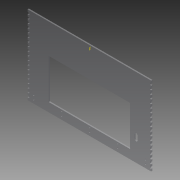
# Autodesk Inventor part: case_front
Saved by Autodesk Inventor 2014 (Build 180170000, 170)
## iProperties
Created: 2013-08-29
Part Number: case_front
Material: Polycarbonate, Clear
Document SubType Name: Modeling
Designer: Edward
Density: 1.2 g/cm^3
Appearance: Polycarbonate - Clear
Author: Edward
Autodesk Inventor part; units mm, degrees
ref_plane "YZ Plane" through (0, 0, 0) normal (1, 0, 0) x (0, 1, 0)
ref_plane "XZ Plane" through (0, 0, 0) normal (0, 1, 0) x (-1, 0, 0)
ref_plane "XY Plane" through (0, 0, 0) normal (0, 0, 1) x (1, 0, 0)
sketch "Sketch1" plane through (0, 0, 0) normal (0, 0, 1) x (1, 0, 0)
  line L0 (303, -45.4136) -> (309.35, -45.4136) projected
  line L1 (303, -45.4136) -> (303, -33.5636) projected
  line L2 (303, 348.2864) -> (309.35, 348.2864) projected
  line L3 (-309.35, 348.2864) -> (-303, 348.2864) projected
  line L4 (-303, -33.5636) -> (-303, -45.4136) projected
  line L5 (303, -45.4136) -> (-303, -45.4136)
  line L6 (-303, -45.4136) -> (-303, 348.2864)
  line L7 (-303, 348.2864) -> (303, 348.2864)
  line L8 (303, 348.2864) -> (303, -45.4136)
  point P0 (0, 0)
  constraints: 8 end point, 2 parallel, 1 horizontal, 1 perpendicular
extrude "Extrusion1" add sketch "Sketch1" along normal blind 6.35
sketch "Sketch3" plane through (303, -45.4136, 0) normal (1, 0, 0) x (0, 0, -1)
  line L0 (0, 393.7) -> (0, 0) projected
  line L1 (-6.35, 0) -> (-6.35, 393.7) projected
  line L2 (0, 21.85) -> (-6.35, 21.85) projected
  line L3 (0, 31.85) -> (-6.35, 31.85) projected
  point P0 (0, 45.4136)
extrude "Extrusion3" add sketch "Sketch3" along normal blind 6.35
pattern_linear "Rectangular Pattern1" count 18 spacing 20 along (0, 1, 0) of "Extrusion3"
sketch "Sketch4" plane through (303, 348.2864, 6.35) normal (1, 0, 0) x (0, 0, -1)
  line L0 (6.35, 0) -> (0, 0) projected
  line L1 (0, -21.85) -> (0, 0) projected
  circle A0 centre (454.35, -377.7) radius 2.75 projected
  circle A1 centre (259.35, -357.7) radius 2.75 projected
  circle A2 centre (64.35, -377.7) radius 2.75 projected
  circle A3 centre (64.35, -357.7) radius 2.75 projected
  circle A4 centre (259.35, -377.7) radius 2.75 projected
  circle A5 centre (454.35, -357.7) radius 2.75 projected
  arc A6 (30.35, -355.2) -> (18.35, -355.2) centre (24.35, -355.2) ccw projected
  line L2 (30.35, -355.2) -> (30.35, -380.2) projected
  arc A7 (18.35, -380.2) -> (30.35, -380.2) centre (24.35, -380.2) ccw projected
  line L3 (18.35, -380.2) -> (18.35, -355.2) projected
  arc A8 (488.35, -380.2) -> (500.35, -380.2) centre (494.35, -380.2) ccw projected
  line L4 (488.35, -380.2) -> (488.35, -355.2) projected
  arc A9 (500.35, -355.2) -> (488.35, -355.2) centre (494.35, -355.2) ccw projected
  line L5 (500.35, -355.2) -> (500.35, -380.2) projected
  line L6 (6.35, -393.7) -> (512.35, -393.7) projected
  line L7 (512.35, -393.7) -> (512.35, -381.85) projected
  line L8 (512.35, -381.85) -> (518.7, -381.85) projected
  line L9 (518.7, -371.85) -> (518.7, -381.85) projected
  line L10 (512.35, -371.85) -> (518.7, -371.85) projected
  line L11 (512.35, -371.85) -> (512.35, -361.85) projected
  line L12 (512.35, -361.85) -> (518.7, -361.85) projected
  line L13 (518.7, -351.85) -> (518.7, -361.85) projected
  line L14 (512.35, -351.85) -> (518.7, -351.85) projected
  line L15 (512.35, -351.85) -> (512.35, -341.85) projected
  line L16 (512.35, -341.85) -> (518.7, -341.85) projected
  line L17 (518.7, -331.85) -> (518.7, -341.85) projected
  line L18 (512.35, -331.85) -> (518.7, -331.85) projected
  line L19 (512.35, -331.85) -> (512.35, -321.85) projected
  line L20 (512.35, -321.85) -> (518.7, -321.85) projected
  line L21 (518.7, -311.85) -> (518.7, -321.85) projected
  line L22 (512.35, -311.85) -> (518.7, -311.85) projected
  line L23 (512.35, -311.85) -> (512.35, -301.85) projected
  line L24 (512.35, -301.85) -> (518.7, -301.85) projected
  line L25 (518.7, -291.85) -> (518.7, -301.85) projected
  line L26 (512.35, -291.85) -> (518.7, -291.85) projected
  line L27 (512.35, -291.85) -> (512.35, -281.85) projected
  line L28 (512.35, -281.85) -> (518.7, -281.85) projected
  line L29 (518.7, -271.85) -> (518.7, -281.85) projected
  line L30 (512.35, -271.85) -> (518.7, -271.85) projected
  line L31 (512.35, -271.85) -> (512.35, -261.85) projected
  line L32 (512.35, -261.85) -> (518.7, -261.85) projected
  line L33 (518.7, -251.85) -> (518.7, -261.85) projected
  line L34 (512.35, -251.85) -> (518.7, -251.85) projected
  line L35 (512.35, -251.85) -> (512.35, -241.85) projected
  line L36 (512.35, -241.85) -> (518.7, -241.85) projected
  line L37 (518.7, -231.85) -> (518.7, -241.85) projected
  line L38 (512.35, -231.85) -> (518.7, -231.85) projected
  line L39 (512.35, -231.85) -> (512.35, -221.85) projected
  line L40 (512.35, -221.85) -> (518.7, -221.85) projected
  line L41 (518.7, -211.85) -> (518.7, -221.85) projected
  line L42 (512.35, -211.85) -> (518.7, -211.85) projected
  line L43 (512.35, -211.85) -> (512.35, -201.85) projected
  line L44 (512.35, -201.85) -> (518.7, -201.85) projected
  line L45 (518.7, -191.85) -> (518.7, -201.85) projected
  line L46 (512.35, -191.85) -> (518.7, -191.85) projected
  line L47 (512.35, -191.85) -> (512.35, -181.85) projected
  line L48 (512.35, -181.85) -> (518.7, -181.85) projected
  line L49 (518.7, -171.85) -> (518.7, -181.85) projected
  line L50 (512.35, -171.85) -> (518.7, -171.85) projected
  line L51 (512.35, -171.85) -> (512.35, -161.85) projected
  line L52 (512.35, -161.85) -> (518.7, -161.85) projected
  line L53 (518.7, -151.85) -> (518.7, -161.85) projected
  line L54 (512.35, -151.85) -> (518.7, -151.85) projected
  line L55 (512.35, -151.85) -> (512.35, -141.85) projected
  line L56 (512.35, -141.85) -> (518.7, -141.85) projected
  line L57 (518.7, -131.85) -> (518.7, -141.85) projected
  line L58 (512.35, -131.85) -> (518.7, -131.85) projected
  line L59 (512.35, -131.85) -> (512.35, -121.85) projected
  line L60 (512.35, -121.85) -> (518.7, -121.85) projected
  line L61 (518.7, -111.85) -> (518.7, -121.85) projected
  line L62 (512.35, -111.85) -> (518.7, -111.85) projected
  line L63 (512.35, -111.85) -> (512.35, -101.85) projected
  line L64 (512.35, -101.85) -> (518.7, -101.85) projected
  line L65 (518.7, -91.85) -> (518.7, -101.85) projected
  line L66 (512.35, -91.85) -> (518.7, -91.85) projected
  line L67 (512.35, -91.85) -> (512.35, -81.85) projected
  line L68 (512.35, -81.85) -> (518.7, -81.85) projected
  line L69 (518.7, -71.85) -> (518.7, -81.85) projected
  line L70 (512.35, -71.85) -> (518.7, -71.85) projected
  line L71 (512.35, -71.85) -> (512.35, -61.85) projected
  line L72 (512.35, -61.85) -> (518.7, -61.85) projected
  line L73 (518.7, -51.85) -> (518.7, -61.85) projected
  line L74 (512.35, -51.85) -> (518.7, -51.85) projected
  line L75 (512.35, -51.85) -> (512.35, -41.85) projected
  line L76 (512.35, -41.85) -> (518.7, -41.85) projected
  line L77 (518.7, -31.85) -> (518.7, -41.85) projected
  line L78 (512.35, -31.85) -> (518.7, -31.85) projected
  line L79 (512.35, -31.85) -> (512.35, -21.85) projected
  line L80 (512.35, -21.85) -> (518.7, -21.85) projected
  line L81 (518.7, -11.85) -> (518.7, -21.85) projected
  line L82 (512.35, -11.85) -> (518.7, -11.85) projected
  line L83 (512.35, -11.85) -> (512.35, 0) projected
  line L84 (100.7265, 0) -> (90.7265, 0) projected
  line L85 (6.35, 0) -> (6.35, -11.85) projected
  line L86 (6.35, -11.85) -> (0, -11.85) projected
  line L87 (0, -21.85) -> (0, -11.85) projected
  line L88 (6.35, -21.85) -> (0, -21.85) projected
  line L89 (6.35, -21.85) -> (6.35, -31.85) projected
  line L90 (6.35, -31.85) -> (0, -31.85) projected
  line L91 (0, -41.85) -> (0, -31.85) projected
  line L92 (6.35, -41.85) -> (0, -41.85) projected
  line L93 (6.35, -41.85) -> (6.35, -51.85) projected
  line L94 (6.35, -51.85) -> (0, -51.85) projected
  line L95 (0, -61.85) -> (0, -51.85) projected
  line L96 (6.35, -61.85) -> (0, -61.85) projected
  line L97 (6.35, -61.85) -> (6.35, -71.85) projected
  line L98 (6.35, -71.85) -> (0, -71.85) projected
  line L99 (0, -81.85) -> (0, -71.85) projected
  line L100 (6.35, -81.85) -> (0, -81.85) projected
  line L101 (6.35, -81.85) -> (6.35, -91.85) projected
  line L102 (6.35, -91.85) -> (0, -91.85) projected
  line L103 (0, -101.85) -> (0, -91.85) projected
  line L104 (6.35, -101.85) -> (0, -101.85) projected
  line L105 (6.35, -101.85) -> (6.35, -111.85) projected
  line L106 (6.35, -111.85) -> (0, -111.85) projected
  line L107 (0, -121.85) -> (0, -111.85) projected
  line L108 (6.35, -121.85) -> (0, -121.85) projected
  line L109 (6.35, -121.85) -> (6.35, -131.85) projected
  line L110 (6.35, -131.85) -> (0, -131.85) projected
  line L111 (0, -141.85) -> (0, -131.85) projected
  line L112 (6.35, -141.85) -> (0, -141.85) projected
  line L113 (6.35, -141.85) -> (6.35, -151.85) projected
  line L114 (6.35, -151.85) -> (0, -151.85) projected
  line L115 (0, -161.85) -> (0, -151.85) projected
  line L116 (6.35, -161.85) -> (0, -161.85) projected
  line L117 (6.35, -161.85) -> (6.35, -171.85) projected
  line L118 (6.35, -171.85) -> (0, -171.85) projected
  line L119 (0, -181.85) -> (0, -171.85) projected
  line L120 (6.35, -181.85) -> (0, -181.85) projected
  line L121 (6.35, -181.85) -> (6.35, -191.85) projected
  line L122 (6.35, -191.85) -> (0, -191.85) projected
  line L123 (0, -201.85) -> (0, -191.85) projected
  line L124 (6.35, -201.85) -> (0, -201.85) projected
  line L125 (6.35, -201.85) -> (6.35, -211.85) projected
  line L126 (6.35, -211.85) -> (0, -211.85) projected
  line L127 (0, -221.85) -> (0, -211.85) projected
  line L128 (6.35, -221.85) -> (0, -221.85) projected
  line L129 (6.35, -221.85) -> (6.35, -231.85) projected
  line L130 (6.35, -231.85) -> (0, -231.85) projected
  line L131 (0, -241.85) -> (0, -231.85) projected
  line L132 (6.35, -241.85) -> (0, -241.85) projected
  line L133 (6.35, -241.85) -> (6.35, -251.85) projected
  line L134 (6.35, -251.85) -> (0, -251.85) projected
  line L135 (0, -261.85) -> (0, -251.85) projected
  line L136 (6.35, -261.85) -> (0, -261.85) projected
  line L137 (6.35, -261.85) -> (6.35, -271.85) projected
  line L138 (6.35, -271.85) -> (0, -271.85) projected
  line L139 (0, -281.85) -> (0, -271.85) projected
  line L140 (6.35, -281.85) -> (0, -281.85) projected
  line L141 (6.35, -281.85) -> (6.35, -291.85) projected
  line L142 (6.35, -291.85) -> (0, -291.85) projected
  line L143 (0, -301.85) -> (0, -291.85) projected
  line L144 (6.35, -301.85) -> (0, -301.85) projected
  line L145 (6.35, -301.85) -> (6.35, -311.85) projected
  line L146 (6.35, -311.85) -> (0, -311.85) projected
  line L147 (0, -321.85) -> (0, -311.85) projected
  line L148 (6.35, -321.85) -> (0, -321.85) projected
  line L149 (6.35, -321.85) -> (6.35, -331.85) projected
  line L150 (6.35, -331.85) -> (0, -331.85) projected
  line L151 (0, -341.85) -> (0, -331.85) projected
  line L152 (6.35, -341.85) -> (0, -341.85) projected
  line L153 (6.35, -341.85) -> (6.35, -351.85) projected
  line L154 (6.35, -351.85) -> (0, -351.85) projected
  line L155 (0, -361.85) -> (0, -351.85) projected
  line L156 (6.35, -361.85) -> (0, -361.85) projected
  line L157 (6.35, -361.85) -> (6.35, -371.85) projected
  line L158 (6.35, -371.85) -> (0, -371.85) projected
  line L159 (0, -381.85) -> (0, -371.85) projected
  line L160 (6.35, -381.85) -> (0, -381.85) projected
  line L161 (6.35, -381.85) -> (6.35, -393.7) projected
  line L162 (6.35, -393.7) -> (0, -393.7) projected
  line L163 (0, -393.7) -> (0, -371.85) projected
  line L164 (480.7265, -6.35) -> (480.7265, 0) projected
  line L165 (480.7265, 0) -> (470.7265, 0) projected
  line L166 (470.7265, 0) -> (470.7265, -6.35) projected
  line L167 (470.7265, -6.35) -> (460.7265, -6.35) projected
  line L168 (460.7265, -6.35) -> (460.7265, 0) projected
  line L169 (460.7265, 0) -> (450.7265, 0) projected
  line L170 (450.7265, 0) -> (450.7265, -6.35) projected
  line L171 (450.7265, -6.35) -> (440.7265, -6.35) projected
  line L172 (440.7265, -6.35) -> (440.7265, 0) projected
  line L173 (440.7265, 0) -> (430.7265, 0) projected
  line L174 (430.7265, 0) -> (430.7265, -6.35) projected
  line L175 (430.7265, -6.35) -> (420.7265, -6.35) projected
  line L176 (420.7265, -6.35) -> (420.7265, 0) projected
  line L177 (420.7265, 0) -> (410.7265, 0) projected
  line L178 (410.7265, 0) -> (410.7265, -6.35) projected
  line L179 (410.7265, -6.35) -> (400.7265, -6.35) projected
  line L180 (400.7265, -6.35) -> (400.7265, 0) projected
  line L181 (400.7265, 0) -> (390.7265, 0) projected
  line L182 (390.7265, 0) -> (390.7265, -6.35) projected
  line L183 (390.7265, -6.35) -> (380.7265, -6.35) projected
  line L184 (380.7265, -6.35) -> (380.7265, 0) projected
  line L185 (380.7265, 0) -> (370.7265, 0) projected
  line L186 (370.7265, 0) -> (370.7265, -6.35) projected
  line L187 (370.7265, -6.35) -> (360.7265, -6.35) projected
  line L188 (360.7265, -6.35) -> (360.7265, 0) projected
  line L189 (360.7265, 0) -> (350.7265, 0) projected
  line L190 (350.7265, 0) -> (350.7265, -6.35) projected
  line L191 (350.7265, -6.35) -> (340.7265, -6.35) projected
  line L192 (340.7265, -6.35) -> (340.7265, 0) projected
  line L193 (340.7265, 0) -> (330.7265, 0) projected
  line L194 (330.7265, 0) -> (330.7265, -6.35) projected
  line L195 (330.7265, -6.35) -> (320.7265, -6.35) projected
  line L196 (320.7265, -6.35) -> (320.7265, 0) projected
  line L197 (320.7265, 0) -> (310.7265, 0) projected
  line L198 (310.7265, 0) -> (310.7265, -6.35) projected
  line L199 (310.7265, -6.35) -> (300.7265, -6.35) projected
  line L200 (300.7265, -6.35) -> (300.7265, 0) projected
  line L201 (300.7265, 0) -> (290.7265, 0) projected
  line L202 (290.7265, 0) -> (290.7265, -6.35) projected
  line L203 (290.7265, -6.35) -> (280.7265, -6.35) projected
  line L204 (280.7265, -6.35) -> (280.7265, 0) projected
  line L205 (280.7265, 0) -> (270.7265, 0) projected
  line L206 (270.7265, 0) -> (270.7265, -6.35) projected
  line L207 (270.7265, -6.35) -> (260.7265, -6.35) projected
  line L208 (260.7265, -6.35) -> (260.7265, 0) projected
  line L209 (260.7265, 0) -> (250.7265, 0) projected
  line L210 (250.7265, 0) -> (250.7265, -6.35) projected
  line L211 (250.7265, -6.35) -> (240.7265, -6.35) projected
  line L212 (240.7265, -6.35) -> (240.7265, 0) projected
  line L213 (230.7265, 0) -> (230.7265, -6.35) projected
  line L214 (230.7265, -6.35) -> (220.7265, -6.35) projected
  line L215 (220.7265, -6.35) -> (220.7265, 0) projected
  line L216 (220.7265, 0) -> (210.7265, 0) projected
  line L217 (210.7265, 0) -> (210.7265, -6.35) projected
  line L218 (210.7265, -6.35) -> (200.7265, -6.35) projected
  line L219 (200.7265, -6.35) -> (200.7265, 0) projected
  line L220 (200.7265, 0) -> (190.7265, 0) projected
  line L221 (190.7265, 0) -> (190.7265, -6.35) projected
  line L222 (190.7265, -6.35) -> (180.7265, -6.35) projected
  line L223 (180.7265, -6.35) -> (180.7265, 0) projected
  line L224 (180.7265, 0) -> (170.7265, 0) projected
  line L225 (170.7265, 0) -> (170.7265, -6.35) projected
  line L226 (170.7265, -6.35) -> (160.7265, -6.35) projected
  line L227 (160.7265, -6.35) -> (160.7265, 0) projected
  line L228 (160.7265, 0) -> (150.7265, 0) projected
  line L229 (150.7265, 0) -> (150.7265, -6.35) projected
  line L230 (150.7265, -6.35) -> (140.7265, -6.35) projected
  line L231 (140.7265, -6.35) -> (140.7265, 0) projected
  line L232 (140.7265, 0) -> (130.7265, 0) projected
  line L233 (130.7265, 0) -> (130.7265, -6.35) projected
  line L234 (130.7265, -6.35) -> (120.7265, -6.35) projected
  line L235 (120.7265, -6.35) -> (120.7265, 0) projected
  line L236 (120.7265, 0) -> (110.7265, 0) projected
  line L237 (110.7265, 0) -> (110.7265, -6.35) projected
  line L238 (110.7265, -6.35) -> (100.7265, -6.35) projected
  line L239 (100.7265, -6.35) -> (100.7265, 0) projected
  line L240 (90.7265, 0) -> (90.7265, -6.35) projected
  line L241 (90.7265, -6.35) -> (80.7265, -6.35) projected
  line L242 (80.7265, -6.35) -> (80.7265, 0) projected
  line L243 (80.7265, 0) -> (70.7265, 0) projected
  line L244 (70.7265, 0) -> (70.7265, -6.35) projected
  line L245 (70.7265, -6.35) -> (60.7265, -6.35) projected
  line L246 (60.7265, -6.35) -> (60.7265, 0) projected
  line L247 (60.7265, 0) -> (50.7265, 0) projected
  line L248 (50.7265, 0) -> (50.7265, -6.35) projected
  line L249 (50.7265, -6.35) -> (40.7265, -6.35) projected
  line L250 (40.7265, -6.35) -> (40.7265, 0) projected
  line L251 (40.7265, 0) -> (30.7265, 0) projected
  line L252 (30.7265, 0) -> (30.7265, -6.35) projected
  line L253 (30.7265, -6.35) -> (20.7265, -6.35) projected
  line L254 (20.7265, -6.35) -> (20.7265, 0) projected
  line L255 (512.35, 0) -> (490.7265, 0) projected
  line L256 (490.7265, 0) -> (490.7265, -6.35) projected
  line L257 (490.7265, -6.35) -> (480.7265, -6.35) projected
  line L258 (240.7265, 0) -> (230.7265, 0) projected
  line L259 (20.7265, 0) -> (6.35, 0) projected
  point P0 (6.35, -348.2864)
extrude "Extrusion4" add sketch "Sketch4" along normal blind 6.35 contours L85 L86 L1 L0 | L160 L161 L162 L163
ref_plane "Work Plane1" through (0, 326.4364, 6.35) normal (1, 0, 0) x (0, 0, -1)
mirror "Mirror1" about plane through (0, 326.4364, 6.35) normal (1, 0, 0) of "Extrusion3", "Rectangular Pattern1", "Extrusion4"
sketch "Sketch6" plane through (0, 0, 6.35) normal (0, 0, 1) x (1, 0, 0)
  circle A0 centre (0, -29.4136) radius 2.75 projected
  circle A1 centre (0, -9.4136) radius 2.75 projected
  circle A2 centre (140, -29.4136) radius 2.75 projected
  circle A3 centre (140, -9.4136) radius 2.75 projected
  circle A4 centre (280, -9.4136) radius 2.75 projected
  circle A5 centre (280, -29.4136) radius 2.75 projected
  circle A6 centre (-280, -29.4136) radius 2.75 projected
  circle A7 centre (-280, -9.4136) radius 2.75 projected
  circle A8 centre (-140, -9.4136) radius 2.75 projected
  circle A9 centre (-140, -29.4136) radius 2.75 projected
  point P0 (0, 0)
extrude "Extrusion5" cut sketch "Sketch6" against normal through all
sketch "Sketch7" plane through (0, 0, 6.35) normal (0, 0, 1) x (1, 0, 0)
  line L0 (-203.65, -0.9136) -> (-203.65, 79.5864) projected
  line L1 (203.65, -0.9136) -> (203.65, 79.5864) projected
  line L2 (303, 6.5864) -> (-297, 6.5864) projected
  line L3 (303, 19.2864) -> (-297, 19.2864) projected
  line L4 (203.65, -0.9136) -> (-203.65, -0.9136)
  line L5 (-203.65, -0.9136) -> (-203.65, 199.0864)
  line L6 (-203.65, 199.0864) -> (203.65, 199.0864)
  line L7 (203.65, 199.0864) -> (203.65, -0.9136)
  point P0 (0, 0)
  dimension "d14" = 200
  constraints: 8 end point, 2 parallel, 1 horizontal, 1 perpendicular
  measures "d14" distance of L4.end L5.end
extrude "Extrusion6" cut sketch "Sketch7" against normal blind 6.35
sketch "Sketch8" plane through (0, 0, 6.35) normal (0, 0, 1) x (1, 0, 0)
  line L0 (-303, 56.4364) -> (-309.35, 56.4364) projected
  circle A0 centre (233.65, 75.5864) radius 5 projected
  circle A1 centre (233.65, 55.5864) radius 5 projected
  line L1 (241.65, 55.5864) -> (241.65, 75.5864)
  arc A2 (241.65, 75.5864) -> (225.65, 75.5864) centre (233.65, 75.5864) ccw
  line L2 (225.65, 75.5864) -> (225.65, 55.5864)
  arc A3 (225.65, 55.5864) -> (241.65, 55.5864) centre (233.65, 55.5864) ccw
  line L3 (238.65, 56.4364) -> (238.65, 55.5864)
  line L4 (228.65, 56.4364) -> (228.65, 55.5864)
  point P0 (0, 0)
  constraints: 8 end point, 6 point on circle, 2 centre point, 2 coincident, 2 point on line, 2 tangent
extrude "Extrusion7" cut sketch "Sketch8" against normal through all contours A0 | A1 | A3 L2 A2 L1
body "Solid1"
